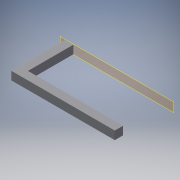
# Autodesk Inventor part: topOfFrame
Saved by Autodesk Inventor 2016 SP1 (Build 200210100, 210)
## iProperties
Created: 2016-01-24
Part Number: topOfFrame
Material: Generic
Document SubType Name: Modeling
Designer: steele
Density: 1 g/cm^3
Appearance: Default
Author: steele
Autodesk Inventor part; units mm, degrees
ref_plane "XZ Plane" through (0, 0, 0) normal (0, 1, 0) x (-1, 0, 0)
sketch "Sketch5" plane through (0, 0, 0) normal (0, 1, 0) x (-1, 0, 0)
  line L0 (0, 0) -> (0, 247.65) construction
  line L1 (0, 0) -> (304.8, 0) construction
  line L2 (0, 247.65) -> (304.8, 247.65)
  line L3 (304.8, 247.65) -> (304.8, 0)
  dimension "d11" = 247.65
  dimension "d12" = 304.8
  constraints: 8 end point, 2 horizontal, 1 perpendicular, 1 vertical
  measures "d11" distance of L0.start L0.end
  measures "d12" distance of L0.start L1.end
sketch "Sketch6" plane through (0, 0, 0) normal (1, 0, 0) x (0, 1, 0)
  line L0 (-12.7, 260.35) -> (-12.7, 234.95)
  line L1 (-12.7, 234.95) -> (12.7, 234.95)
  line L2 (12.7, 234.95) -> (12.7, 260.35)
  line L3 (12.7, 260.35) -> (-12.7, 260.35)
  line L4 (-12.7, 260.35) -> (12.7, 234.95) construction
  line L5 (-12.7, 234.95) -> (12.7, 260.35) construction
  point P0 (0, 0)
  point P1 (0, 247.65)
  dimension "d13" = 25.4
  dimension "d14" = 25.4
  dimension "d15" = 247.65
  constraints: 12 end point, 2 midpoint, 2 parallel, 1 perpendicular, 1 vertical
  measures "d13" distance of L2.end L0.start
  measures "d14" distance of L1.end L2.end
  measures "d15" distance of point (0, 0) point (0, 247.65)
sweep "Sweep2" add profiles "Sketch6" path "Sketch5"
ref_plane "Work Plane1" through (-304.8, 0, 0) normal (1, 0, 0) x (0, 1, 0)
equation "\"d11\" = width"
equation "\"d12\" = length"
equation "\"d15\" = width"
equation "\"width\" = 247.65"
equation "\"length\" = 304.8"
equation "\"d18\" = -length"
equation "\"height\" = 241.3"
body "Solid2"
